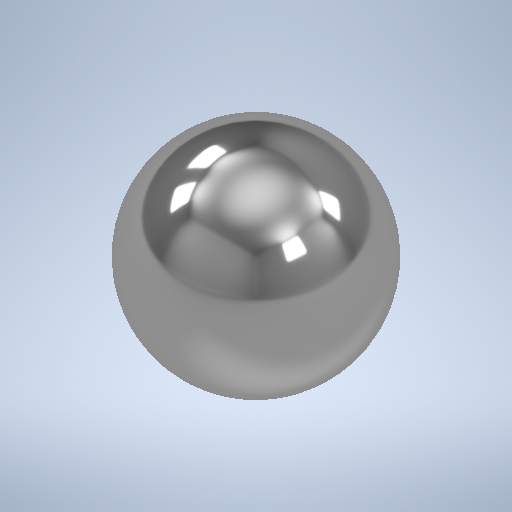
# Autodesk Inventor part: sessao_07_04_004_001
Saved by Autodesk Inventor 2026 (Build 300175000, 175)
## iProperties
Created: 2025-04-07
Part Number: sessao_07_04_004_001
Material: Glass
Document SubType Name: Modeling
Designer: Carlos Dias
Density: 2.18 g/cm^3
Appearance: Chrome - Polished Black
Author: Carlos Dias
Autodesk Inventor part; units mm, degrees
sketch "Sketch1" plane through (0, 0, 0) normal (0, 0, 1) x (1, 0, 0)
  circle A0 centre (0, 0) radius 15 construction
  line L0 (0, 15) -> (0, -15)
  arc A1 (0, 15) -> (0, -15) centre (0, 0) ccw
  dimension "d7" = 30
  dimension "d8" = 30
  constraints: 4 point on circle, 2 centre point, 2 coincident, 2 end point, 1 concentric, 1 vertical
  measures "d7" diameter of A0
  measures "d8" distance of L0.start L0.end
revolve "Revolution1" add sketch "Sketch1" angle 360 about axis through (0, 15, 0) along (0, -1, 0)
body "Solid2"
